Autodesk Fusion 360 part; units mm, degrees
note: some values were not read from the file. Set by a fixed rule: which face or edge a step refers to.
(part 2 of 3)
sketch "Joins" plane through (0, 0, 0) normal (0, 0, 1) x (1, 0, 0)
  line L0 (-32.0183, 52.9002) -> (-40.0183, 52.8995)
  arc A0 (-40.0183, 52.8995) -> (-40.0176, 45.3995) centre (-40.018, 49.1495) ccw
  line L1 (-40.0176, 45.3995) -> (-32.0176, 45.4002)
  arc A1 (-32.0176, 45.4002) -> (-32.0183, 52.9002) centre (-32.018, 49.1502) ccw
  line L2 (-32.018, 49.1502) -> (-40.018, 49.1495) construction
  line L3 (-23.6888, 49.151) -> (-32.018, 49.1502)
  arc A2 (-40.0183, 42.8995) -> (-40.0176, 35.3995) centre (-40.018, 39.1495) ccw
  line L4 (-40.0176, 35.3995) -> (-32.0176, 35.4002)
  arc A3 (-32.0176, 35.4002) -> (-32.0183, 42.9002) centre (-32.018, 39.1502) ccw
  line L5 (-32.0183, 42.9002) -> (-40.0183, 42.8995)
  arc A4 (-32.0176, 25.4002) -> (-32.0183, 32.9002) centre (-32.018, 29.1502) ccw
  line L6 (-32.0183, 32.9002) -> (-40.0183, 32.8995)
  arc A5 (-40.0183, 32.8995) -> (-40.0176, 25.3995) centre (-40.018, 29.1495) ccw
  line L7 (-40.0176, 25.3995) -> (-32.0176, 25.4002)
  arc A6 (-40.0183, 22.8995) -> (-40.0176, 15.3995) centre (-40.018, 19.1495) ccw
  line L8 (-40.0176, 15.3995) -> (-32.0176, 15.4002)
  arc A7 (-32.0176, 15.4002) -> (-32.0183, 22.9002) centre (-32.018, 19.1502) ccw
  line L9 (-32.0183, 22.9002) -> (-40.0183, 22.8995)
  arc A8 (-40.0183, 12.8995) -> (-40.0176, 5.3995) centre (-40.018, 9.1495) ccw
  line L10 (-40.0176, 5.3995) -> (-32.0176, 5.4002)
  arc A9 (-32.0176, 5.4002) -> (-32.0183, 12.9002) centre (-32.018, 9.1502) ccw
  line L11 (-32.0183, 12.9002) -> (-40.0183, 12.8995)
  arc A10 (11.7309, 47.7843) -> (11.9097, 40.2864) centre (11.8203, 44.0353) ccw
  line L12 (11.9097, 40.2864) -> (19.9074, 40.4771)
  arc A11 (19.9074, 40.4771) -> (19.7286, 47.975) centre (19.818, 44.2261) ccw
  line L13 (19.7286, 47.975) -> (11.7309, 47.7843)
  line L14 (11.9129, 30.2801) -> (19.9104, 30.4772)
  arc A12 (19.9104, 30.4772) -> (19.7256, 37.9749) centre (19.818, 34.2261) ccw
  arc A13 (11.7281, 37.7778) -> (11.9129, 30.2801) centre (11.8205, 34.029) ccw
  line L15 (19.7256, 37.9749) -> (11.7281, 37.7778)
  line L16 (11.8351, 20.44) -> (19.835, 20.4761)
  arc A14 (19.835, 20.4761) -> (19.8011, 27.976) centre (19.818, 24.2261) ccw
  arc A15 (11.8012, 27.9399) -> (11.8351, 20.44) centre (11.8181, 24.1899) ccw
  line L17 (19.8011, 27.976) -> (11.8012, 27.9399)
  point P0 (-32.018, 49.1502)
  dimension "d51" = 8
  dimension "d52" = 7.5
  dimension "d53" = 8
  dimension "d54" = 7.5
  dimension "d55" = 8
  dimension "d56" = 7.5
  dimension "d57" = 8
  dimension "d58" = 7.5
  dimension "d59" = 8
  dimension "d60" = 7.5
  dimension "d61" = 8
  dimension "d62" = 7.5
  dimension "d63" = 8
  dimension "d64" = 7.5
  dimension "d65" = 8
  dimension "d66" = 7.5
  constraint tangent L0 A0
  constraint tangent A0 L1
  constraint parallel L0 L1
  constraint tangent L1 A1
  constraint tangent L0 A1
  constraint parallel L2 L3
  constraint coincident P0 A1.centre
  constraint tangent A2 L5
  constraint tangent A2 L4
  constraint parallel L4 L5
  constraint tangent L4 A3
  constraint tangent A3 L5
  constraint tangent L6 A5
  constraint tangent A5 L7
  constraint parallel L6 L7
  constraint tangent A4 L7
  constraint tangent A4 L6
  constraint tangent A6 L9
  constraint tangent A6 L8
  constraint parallel L8 L9
  constraint tangent L8 A7
  constraint tangent A7 L9
  constraint tangent A8 L11
  constraint tangent A8 L10
  constraint parallel L10 L11
  constraint tangent L10 A9
  constraint tangent A9 L11
  constraint tangent A10 L13
  constraint tangent A10 L12
  constraint parallel L12 L13
  constraint tangent L12 A11
  constraint tangent A11 L13
  constraint tangent A13 L15
  constraint tangent L14 A13
  constraint parallel L14 L15
  constraint tangent L14 A12
  constraint tangent A12 L15
  constraint tangent A15 L17
  constraint tangent L16 A15
  constraint parallel L16 L17
  constraint tangent L16 A14
  constraint tangent A14 L17
  measures "d51" distance of P0 A0.centre
  measures "d52" diameter of A0
  measures "d53" distance of A2.centre A3.centre
  measures "d54" diameter of A2
  measures "d55" distance of A5.centre A4.centre
  measures "d56" diameter of A5
  measures "d57" distance of A6.centre A7.centre
  measures "d58" diameter of A6
  measures "d59" distance of A8.centre A9.centre
  measures "d60" diameter of A8
  measures "d61" distance of A10.centre A11.centre
  measures "d62" diameter of A10
  measures "d63" distance of A13.centre A12.centre
  measures "d64" diameter of A13
  measures "d65" distance of A15.centre A14.centre
  measures "d66" diameter of A15
extrude "Extrude8" cut sketch "Joins" against normal blind 2.7 bodies 1
extrude "Extrude9" add sketch "Joins" along normal blind 4 separate body makes body 19 at (-34.6848, 40.4, 0) makes body 20 at (-34.6848, 20.4, 0) makes body 21 at (17.1819, 42.9128, 0) makes body 22 at (-34.6848, 30.4, 0) makes body 23 at (-37.3512, 47.8997, 4) makes body 24 at (-34.6848, 10.4, 0) makes body 25 at (17.1214, 35.41, 0) makes body 26 at (17.1458, 25.464, 0)
move_body "Move4" bodies 22 23 24 21 25 20 26 19 to x (1, 0, 0) y (0, 1, 0) z (0, 0, 1) at (0, 0, -8.7)
combine "Combine5" operation cut target body 1 tool bodies 19 22 25 20 23 24 26 21
sketch "Border" plane through (0, 0, 0) normal (0, 0, 1) x (-1, 0, 0)
  line L0 (101.7185, 44.7509) -> (-98.6412, 44.7509)
  line L1 (-98.6412, 44.7509) -> (-98.6412, -80.6951)
  line L2 (-98.6412, -80.6951) -> (101.7185, -80.6951)
  line L3 (101.7185, -80.6951) -> (101.7185, 44.7509)
  arc A0 (32.0176, -5.4002) -> (28.6259, -7.5514) centre (32.018, -9.1502) ccw
  line L4 (32.0176, -5.4002) -> (40.0176, -5.3995)
  arc A1 (40.0183, -12.8995) -> (40.0176, -5.3995) centre (40.018, -9.1495) ccw
  line L5 (40.0183, -12.8995) -> (32.0183, -12.9002)
  arc A2 (28.6396, -10.7778) -> (32.0183, -12.9002) centre (32.018, -9.1502) ccw
  line L6 (28.6396, -10.7778) -> (26.121, -10.7778)
  line L7 (26.121, -10.7778) -> (26.121, -18.6304)
  arc A3 (24.5959, -20.7696) -> (26.121, -18.6304) centre (24.596, -19.1564) ccw
  line L8 (24.5959, -20.7696) -> (17.0179, -20.7691)
  line L9 (16.4913, -20.6807) -> (2.5732, -20.6743)
  arc A4 (2.5746, -17.6243) -> (2.5732, -20.6743) centre (2.5739, -19.1493) ccw
  line L10 (2.5746, -17.6243) -> (16.4927, -17.6307)
  line L11 (17.0181, -17.5428) -> (23.071, -17.5432)
  line L12 (23.071, -17.5432) -> (23.071, -9.6906)
  arc A5 (24.596, -7.5514) -> (23.071, -9.6906) centre (24.596, -9.1646) ccw
  line L13 (24.596, -7.5514) -> (28.6259, -7.5514)
  circle A6 centre (1.524, -36.656) radius 0.45
  circle A7 centre (17.018, -6.656) radius 0.45
  circle A8 centre (9.271, -0.998) radius 0.45
  circle A9 centre (17.018, -31.656) radius 0.45
  circle A10 centre (17.018, -34.156) radius 0.45
  circle A11 centre (17.018, -9.156) radius 0.45
  circle A12 centre (17.018, -16.656) radius 0.45
  circle A13 centre (1.524, -6.656) radius 0.45
  circle A14 centre (17.018, -26.656) radius 0.45
  circle A15 centre (1.524, -21.656) radius 0.45
  circle A16 centre (1.524, -26.656) radius 0.45
  circle A17 centre (1.524, -9.156) radius 0.45
  circle A18 centre (1.524, -16.656) radius 0.45
  circle A19 centre (9.271, -3) radius 0.45
  circle A20 centre (7.271, -0.9961) radius 0.45
  circle A21 centre (17.018, -4.156) radius 0.45
  circle A22 centre (1.524, -4.156) radius 0.45
  circle A23 centre (11.269, -3) radius 0.45
  circle A24 centre (1.524, -31.656) radius 0.45
  circle A25 centre (1.524, -11.656) radius 0.45
  circle A26 centre (17.018, -21.656) radius 0.45
  circle A27 centre (17.018, -11.656) radius 0.45
  circle A28 centre (17.018, -14.156) radius 0.45
  circle A29 centre (17.018, -36.656) radius 0.45
  circle A30 centre (11.2599, -1.0002) radius 0.45
  circle A31 centre (7.271, -3.0017) radius 0.45
  arc A32 (40.0183, -22.8995) -> (40.0176, -15.3995) centre (40.018, -19.1495) ccw
  line L14 (40.0183, -22.8995) -> (32.0183, -22.9002)
  arc A33 (32.0176, -15.4002) -> (32.0183, -22.9002) centre (32.018, -19.1502) ccw
  line L15 (32.0176, -15.4002) -> (40.0176, -15.3995)
  arc A34 (-11.7309, -47.7843) -> (-11.9097, -40.2864) centre (-11.8203, -44.0353) ccw
  line L16 (-11.7309, -47.7843) -> (-19.7286, -47.975)
  arc A35 (-19.9074, -40.4771) -> (-19.7286, -47.975) centre (-19.818, -44.2261) ccw
  line L17 (-19.9074, -40.4771) -> (-11.9097, -40.2864)
  line L18 (40.0183, -52.8995) -> (32.0183, -52.9002)
  arc A36 (32.0176, -45.4002) -> (32.0183, -52.9002) centre (32.018, -49.1502) ccw
  line L19 (32.0176, -45.4002) -> (40.0176, -45.3995)
  arc A37 (40.0183, -52.8995) -> (40.0176, -45.3995) centre (40.018, -49.1495) ccw
  arc A38 (28.594, -40.6795) -> (32.0183, -42.9002) centre (32.018, -39.1502) ccw
  line L20 (28.594, -40.6795) -> (17.0182, -40.681)
  arc A39 (17.0041, -40.681) -> (17.0182, -40.681) centre (17.018, -39.156) ccw
  line L21 (17.0041, -40.681) -> (1.6701, -40.6778)
  arc A40 (1.6707, -37.6278) -> (1.6701, -40.6778) centre (1.6704, -39.1528) ccw
  line L22 (1.6707, -37.6278) -> (17.0047, -37.631)
  arc A41 (17.0178, -37.6309) -> (17.0047, -37.631) centre (17.018, -39.156) ccw
  line L23 (17.0178, -37.6309) -> (28.5902, -37.6293)
  arc A42 (32.0176, -35.4002) -> (28.5902, -37.6293) centre (32.018, -39.1502) ccw
  line L24 (32.0176, -35.4002) -> (40.0176, -35.3995)
  arc A43 (40.0183, -42.8995) -> (40.0176, -35.3995) centre (40.018, -39.1495) ccw
  line L25 (40.0183, -42.8995) -> (32.0183, -42.9002)
  arc A44 (-8.4113, -22.6228) -> (-11.8351, -20.44) centre (-11.8181, -24.1899) ccw
  line L26 (-8.4113, -22.6228) -> (1.6713, -22.6262)
  line L27 (1.6713, -22.6262) -> (17.0185, -22.631)
  arc A45 (17.0175, -25.681) -> (17.0185, -22.631) centre (17.018, -24.156) ccw
  line L28 (17.0175, -25.681) -> (1.6704, -25.6762)
  line L29 (1.6704, -25.6762) -> (-8.3738, -25.6728)
  line L30 (-11.8012, -27.9399) -> (-19.8011, -27.976)
  arc A46 (-19.835, -20.4761) -> (-19.8011, -27.976) centre (-19.818, -24.2261) ccw
  line L31 (-19.835, -20.4761) -> (-11.8351, -20.44)
  arc A47 (28.596, -30.684) -> (32.0183, -32.9002) centre (32.018, -29.1502) ccw
  line L32 (28.596, -30.684) -> (17.0369, -30.6809)
  arc A48 (17.0176, -30.681) -> (17.0369, -30.6809) centre (17.018, -29.156) ccw
  line L33 (17.0176, -30.681) -> (1.6701, -30.6768)
  arc A49 (1.671, -27.6268) -> (1.6701, -30.6768) centre (1.6705, -29.1518) ccw
  line L34 (1.671, -27.6268) -> (17.0184, -27.631)
  arc A50 (17.0377, -27.6311) -> (17.0184, -27.631) centre (17.018, -29.156) ccw
  line L35 (17.0377, -27.6311) -> (28.5881, -27.6343)
  arc A51 (32.0176, -25.4002) -> (28.5881, -27.6343) centre (32.018, -29.1502) ccw
  line L36 (32.0176, -25.4002) -> (40.0176, -25.3995)
  arc A52 (40.0183, -32.8995) -> (40.0176, -25.3995) centre (40.018, -29.1495) ccw
  line L37 (40.0183, -32.8995) -> (32.0183, -32.9002)
  arc A53 (-8.3422, -32.6274) -> (-11.9129, -30.2801) centre (-11.8205, -34.029) ccw
  line L38 (-8.3422, -32.6274) -> (1.6714, -32.6293)
  line L39 (1.6714, -32.6293) -> (11.7302, -32.631)
  arc A54 (13.1178, -34.7881) -> (11.7302, -32.631) centre (11.73, -34.156) ccw
  arc A55 (10.226, -35.6807) -> (13.1178, -34.7881) centre (11.7277, -35.4153) ccw
  line L40 (10.226, -35.6807) -> (1.6709, -35.6793)
  line L41 (1.6709, -35.6793) -> (-8.4522, -35.6774)
  line L42 (-11.7281, -37.7778) -> (-19.7256, -37.9749)
  arc A56 (-19.9104, -30.4772) -> (-19.7256, -37.9749) centre (-19.818, -34.2261) ccw
  line L43 (-19.9104, -30.4772) -> (-11.9129, -30.2801)
  line L44 (-6.5778, -60.1235) -> (22.1197, -60.1235)
  line L45 (39.1197, -43.1235) -> (39.1197, -2.2457)
  line L46 (26.1197, 10.7543) -> (-6.5778, 10.7543)
  line L47 (-19.5778, -2.2457) -> (-19.5778, -47.1235)
  arc A57 (22.1197, -60.1235) -> (39.1197, -43.1235) centre (22.1197, -43.1235) ccw
  arc A58 (-19.5778, -47.1235) -> (-6.5778, -60.1235) centre (-6.5778, -47.1235) ccw
  arc A59 (39.1197, -2.2457) -> (26.1197, 10.7543) centre (26.1197, -2.2457) ccw
  arc A60 (-6.5778, 10.7543) -> (-19.5778, -2.2457) centre (-6.5778, -2.2457) ccw
  arc A61 (16.4913, -20.6807) -> (17.0179, -20.7691) centre (17.018, -19.156) ccw
  arc A62 (17.0181, -17.5428) -> (16.4927, -17.6307) centre (17.018, -19.156) ccw
  arc A63 (-11.8012, -27.9399) -> (-8.3738, -25.6728) centre (-11.8181, -24.1899) ccw
  arc A64 (-11.7281, -37.7778) -> (-8.4522, -35.6774) centre (-11.8205, -34.029) ccw
  circle A65 centre (1.524, -14.156) radius 0.45
  point P0 (9.271, -24.6846)
  dimension "d76" = 17
  dimension "d77" = 13
  constraint horizontal L44
  constraint perpendicular L44 L45
  constraint parallel L44 L46
  constraint parallel L45 L47
  constraint tangent L45 A57
  constraint tangent L44 A57
  constraint tangent L44 A58
  constraint tangent L47 A58
  constraint tangent L46 A59
  constraint tangent L45 A59
  constraint equal A58 A59
  constraint tangent L46 A60
  constraint tangent L47 A60
  constraint equal A58 A60
  measures "d76" radius of A57
  measures "d77" radius of A58
extrude "Extrude10" cut sketch "Border" against normal blind 8.7 contours A0 L4 L5 A2 L6 L7 A3 L8 L9 A4 L10 L11 L12 A5 L13 L45 A61 A62 | A0 L4 L5 A2 L6 L7 A3 L8 L9 A4 L10 L11 L12 A5 L13 L14 A33 L15 A34 L16 L17 L18 A36 L19 A38 L20 A39 L21 A40 L22 A41 L23 A42 L24 L25 A44 L26 L27 A45 L28 L29 L30 L31 A47 L32 A48 L33 A49 L34 A50 L35 A51 L36 L37 A53 L38 L39 A54 A55 L40 L41 L42 L43 L44 L45 L46 L47 A57 A58 A59 A60 A61 A62 A63 A64 | L4 A1 L5 L45 | L14 A33 L15 L45 | A32 L14 L15 L45 | A47 L32 A48 L33 A49 L34 A50 L35 A51 L36 L37 L45 | L36 A52 L37 L45 | L30 A46 L31 L47 | A44 L26 L27 A45 L28 L29 L30 L31 L47 A63 | A38 L20 A39 L21 A40 L22 A41 L23 A42 L24 L25 L45 | L24 A43 L25 L45 | L42 A56 L43 L47 | A53 L38 L39 A54 A55 L40 L41 L42 L43 L47 A64 | L18 A36 L19 A57 | L18 L19 A37 A57 | L16 A35 L17 L47 A58 | A34 L16 L17 L47 A58 | A6 | A7 | A8 | A9 | A10 | A11 | A12 | A13 | A14 | A15 | A16 | A17 | A18 | A19 | A20 | A21 | A22 | A23 | A24 | A25 | A26 | A27 | A28 | A29 | A30 | A31 | A65 keep common part bodies 1
sketch "ArduinoExtrusion" plane through (0, 0, 0) normal (0, 0, 1) x (1, 0, 0)
  line L0 (-18.542, 0) -> (0, 0)
  line L1 (0, 0) -> (0, 43.18)
  line L2 (0, 43.18) -> (-18.542, 43.18)
  line L3 (-18.542, 43.18) -> (-18.542, 0)
  line L4 (-15.829, 4.2) -> (-2.8014, 4.2)
  line L5 (-2.8014, 4.2) -> (-2.8014, 43.18)
  line L6 (-2.8014, 43.18) -> (-15.829, 43.18)
  line L7 (-15.829, 43.18) -> (-15.829, 4.2)
  line L8 (-15.829, 43.18) -> (-2.8014, 43.18)
  line L9 (-2.8014, 43.18) -> (-2.8014, 65.9759)
  line L10 (-2.8014, 65.9759) -> (-15.829, 65.9759)
  line L11 (-15.829, 65.9759) -> (-15.829, 43.18)
  line L12 (-19.542, -1) -> (1, -1)
  line L13 (1, -1) -> (1, 44.18)
  line L14 (1, 44.18) -> (-19.542, 44.18)
  line L15 (-19.542, 44.18) -> (-19.542, -1)
  point P0 (-18.542, 0)
  point P1 (0, 43.18)
  point P2 (-15.829, 4.2)
  point P3 (-2.8014, 43.18)
  dimension "d92" = 1
  constraint horizontal L0
  constraint vertical L1
  constraint horizontal L2
  constraint vertical L3
  constraint coincident P1 L1.end
  constraint coincident P0 L0.start
  constraint horizontal L4
  constraint vertical L5
  constraint horizontal L6
  constraint vertical L7
  constraint coincident P3 L5.end
  constraint coincident P2 L4.start
  constraint horizontal L8
  constraint vertical L9
  constraint horizontal L10
  constraint vertical L11
extrude "Extrude12" cut sketch "ArduinoExtrusion" against normal blind 0.2 contours L2 L6 L8 L9 L11 L14 | L9 L10 L11 L14 bodies 1
extrude "Extrude13" cut sketch "ArduinoExtrusion" against normal blind 1.2 contours L0 L1 L2 L3 L4 L5 L7 | L0 L1 L2 L3 L9 L11 L12 L13 L14 L15 | L2 L6 L8 L9 L11 L14 | L2 L4 L5 L6 L7 L8 bodies 1
sketch "PaintJointsHole" plane through (0, 0, 0) normal (0, 0, 1) x (1, 0, 0)
  circle A0 centre (-32.018, 49.1502) radius 1.525
  circle A1 centre (-32.018, 39.1502) radius 1.525
  circle A2 centre (-32.018, 29.1502) radius 1.525
  circle A3 centre (-32.018, 19.1502) radius 1.525
  circle A4 centre (-32.018, 9.1502) radius 1.525
  circle A5 centre (11.8181, 24.1899) radius 1.525
  circle A6 centre (11.8205, 34.029) radius 1.525
  circle A7 centre (11.8203, 44.0353) radius 1.525
  point P0 (-32.018, 49.1502)
  point P1 (-32.018, 39.1502)
  point P2 (-32.018, 29.1502)
  point P3 (-32.018, 19.1502)
  point P4 (-32.018, 9.1502)
  point P5 (11.5344, 13.9344)
  point P6 (11.8181, 24.1899)
  point P7 (11.8205, 34.029)
  point P8 (11.8203, 44.0353)
  dimension "d88" = 3.05
  constraint coincident P0 A0.centre
  constraint coincident P1 A1.centre
  constraint coincident P2 A2.centre
  constraint coincident P3 A3.centre
  constraint coincident P4 A4.centre
  constraint coincident P6 A5.centre
  constraint coincident P7 A6.centre
  constraint coincident P8 A7.centre
  constraint equal A0 A1
  constraint equal A0 A2
  constraint equal A0 A7
  constraint equal A0 A6
  constraint equal A0 A5
  constraint equal A0 A3
  constraint equal A0 A4
  measures "d88" diameter of A0
extrude "Extrude15" cut sketch "PaintJointsHole" against normal blind 8.7 bodies 1
sketch "CutBetweenLeg" plane through (0, 0, 0) normal (0, 0, 1) x (1, 0, 0)
  line L0 (-39.1197, 35.6745) -> (-53.3111, 35.6745)
  arc A0 (-53.3111, 35.6745) -> (-53.3111, 32.6245) centre (-53.3111, 34.1495) ccw
  line L1 (-53.3111, 32.6245) -> (-39.1197, 32.6245)
  arc A1 (-39.1197, 32.6245) -> (-39.1197, 35.6745) centre (-39.1197, 34.1495) ccw
  line L2 (-39.1197, 34.1495) -> (-53.3111, 34.1495) construction
  line L3 (-39.1197, 32.8995) -> (-39.1197, 35.3995)
  line L4 (-39.0814, 45.7891) -> (-53.3111, 45.7891)
  arc A2 (-53.3111, 45.7891) -> (-53.3111, 42.7391) centre (-53.3111, 44.2641) ccw
  line L5 (-53.3111, 42.7391) -> (-39.0814, 42.7391)
  arc A3 (-39.0814, 42.7391) -> (-39.0814, 45.7891) centre (-39.0814, 44.2641) ccw
  line L6 (-39.0814, 44.2641) -> (-53.3111, 44.2641) construction
  arc A4 (-38.9667, 45.3996) -> (-39.1197, 43.1235) centre (-22.1197, 43.1235) ccw
  line L7 (-39.1197, 25.6745) -> (-53.3111, 25.6745)
  arc A5 (-53.3111, 25.6745) -> (-53.3111, 22.6245) centre (-53.3111, 24.1495) ccw
  line L8 (-53.3111, 22.6245) -> (-39.1197, 22.6245)
  arc A6 (-39.1197, 22.6245) -> (-39.1197, 25.6745) centre (-39.1197, 24.1495) ccw
  line L9 (-39.1197, 24.1495) -> (-53.3111, 24.1495) construction
  line L10 (-39.1197, 22.8995) -> (-39.1197, 25.3995)
  line L11 (-39.1197, 15.6745) -> (-53.3111, 15.6745)
  arc A7 (-53.3111, 15.6745) -> (-53.3111, 12.6245) centre (-53.3111, 14.1495) ccw
  line L12 (-53.3111, 12.6245) -> (-39.1197, 12.6245)
  arc A8 (-39.1197, 12.6245) -> (-39.1197, 15.6745) centre (-39.1197, 14.1495) ccw
  line L13 (-39.1197, 14.1495) -> (-53.3111, 14.1495) construction
  line L14 (-39.1197, 12.8995) -> (-39.1197, 15.3995)
  line L15 (19.5778, 20.4749) -> (19.5778, 2.2457)
  line L16 (19.5778, 27.697) -> (37.3869, 27.697)
  arc A9 (37.3869, 27.697) -> (37.3869, 30.747) centre (37.3869, 29.222) ccw
  line L17 (37.3869, 30.747) -> (19.5778, 30.747)
  arc A10 (19.5778, 30.747) -> (19.5778, 27.697) centre (19.5778, 29.222) ccw
  line L18 (19.5778, 29.222) -> (37.3869, 29.222) construction
  line L19 (19.5778, 30.469) -> (19.5778, 27.975)
  line L20 (19.5778, 37.6953) -> (37.3869, 37.6953)
  arc A11 (37.3869, 37.6953) -> (37.3869, 40.7453) centre (37.3869, 39.2203) ccw
  line L21 (37.3869, 40.7453) -> (19.5778, 40.7453)
  arc A12 (19.5778, 40.7453) -> (19.5778, 37.6953) centre (19.5778, 39.2203) ccw
  line L22 (19.5778, 39.2203) -> (37.3869, 39.2203) construction
  line L23 (19.5778, 40.4693) -> (19.5778, 37.9713)
  dimension "d108" = 3.05
  dimension "d109" = 3.05
  dimension "d110" = 3.05
  dimension "d111" = 3.05
  dimension "d113" = 3.05
  dimension "d114" = 3.05
  constraint tangent L0 A0
  constraint tangent A0 L1
  constraint parallel L0 L1
  constraint tangent L1 A1
  constraint tangent L0 A1
  constraint perpendicular L2 L3
  constraint midpoint A1.centre L3
  constraint tangent L4 A2
  constraint tangent A2 L5
  constraint parallel L4 L5
  constraint tangent L5 A3
  constraint tangent L4 A3
  constraint parallel L0 L6
  constraint midpoint A3.centre A4
  constraint tangent L7 A5
  constraint tangent A5 L8
  constraint parallel L7 L8
  constraint tangent L8 A6
  constraint tangent L7 A6
  constraint perpendicular L3 L9
  constraint midpoint A6.centre L10
  constraint tangent L11 A7
  constraint tangent A7 L12
  constraint parallel L11 L12
  constraint tangent L12 A8
  constraint tangent L11 A8
  constraint perpendicular L13 L14
  constraint midpoint A8.centre L14
  constraint tangent L16 A9
  constraint tangent A9 L17
  constraint parallel L16 L17
  constraint tangent L17 A10
  constraint tangent L16 A10
  constraint perpendicular L18 L19
  constraint midpoint A10.centre L19
  constraint tangent L20 A11
  constraint tangent A11 L21
  constraint parallel L20 L21
  constraint tangent L21 A12
  constraint tangent L20 A12
  constraint perpendicular L22 L23
  constraint midpoint A12.centre L23
  measures "d108" diameter of A0
  measures "d109" diameter of A2
  measures "d110" diameter of A5
  measures "d111" diameter of A7
  measures "d113" diameter of A9
  measures "d114" diameter of A11
extrude "Extrude17" cut sketch "CutBetweenLeg" against normal blind 8.7 bodies 1
sketch "Sketch20" plane through (0, 0, 0) normal (0, 0, 1) x (1, 0, 0)
  line L0 (21.2354, 40.7542) -> (19.5778, 40.7508)
  line L1 (19.5778, 37.7008) -> (21.2402, 37.6959)
  arc A0 (18.7043, 37.9757) -> (19.5778, 37.7008) centre (19.5778, 39.2258) ccw
  arc A1 (18.7041, 40.4757) -> (18.7043, 37.9757) centre (19.5778, 39.2258) ccw
  arc A2 (19.5778, 40.7508) -> (18.7041, 40.4757) centre (19.5778, 39.2258) ccw
  line L2 (21.2434, 20.7575) -> (19.5778, 20.7508)
  line L3 (19.5778, 17.7008) -> (21.251, 17.6915)
  arc A3 (18.7043, 17.9757) -> (19.5778, 17.7008) centre (19.5778, 19.2258) ccw
  arc A4 (18.7041, 20.4757) -> (18.7043, 17.9757) centre (19.5778, 19.2258) ccw
  arc A5 (19.5778, 20.7508) -> (18.7041, 20.4757) centre (19.5778, 19.2258) ccw
  line L4 (-41.123, 42.732) -> (-39.0815, 42.7388)
  arc A6 (-38.0632, 45.3991) -> (-39.0815, 45.7888) centre (-39.0815, 44.2638) ccw
  arc A7 (-38.401, 42.899) -> (-38.0632, 45.3991) centre (-39.0815, 44.2638) ccw
  arc A8 (-39.0815, 42.7388) -> (-38.401, 42.899) centre (-39.0815, 44.2638) ccw
  line L5 (-39.0815, 45.7888) -> (-41.6972, 45.7955)
  line L6 (-41.4536, 12.6128) -> (-39.1197, 12.624)
  line L7 (-39.1197, 15.674) -> (-41.4536, 15.6842)
  arc A9 (-38.2463, 15.3991) -> (-39.1197, 15.674) centre (-39.1197, 14.149) ccw
  arc A10 (-38.2461, 12.8991) -> (-38.2463, 15.3991) centre (-39.1197, 14.149) ccw
  arc A11 (-39.1197, 12.624) -> (-38.2461, 12.8991) centre (-39.1197, 14.149) ccw
  line L8 (-41.4513, 22.6138) -> (-39.1197, 22.624)
  line L9 (-39.1197, 25.674) -> (-41.4504, 25.6829)
  arc A12 (-38.2463, 25.3991) -> (-39.1197, 25.674) centre (-39.1197, 24.149) ccw
  arc A13 (-38.2461, 22.8991) -> (-38.2463, 25.3991) centre (-39.1197, 24.149) ccw
  arc A14 (-39.1197, 22.624) -> (-38.2461, 22.8991) centre (-39.1197, 24.149) ccw
  line L10 (21.2387, 30.7556) -> (19.5778, 30.7508)
  line L11 (19.5778, 27.7008) -> (21.245, 27.694)
  arc A15 (18.7043, 27.9757) -> (19.5778, 27.7008) centre (19.5778, 29.2258) ccw
  arc A16 (18.7041, 30.4757) -> (18.7043, 27.9757) centre (19.5778, 29.2258) ccw
  arc A17 (19.5778, 30.7508) -> (18.7041, 30.4757) centre (19.5778, 29.2258) ccw
  line L12 (-41.4481, 32.6151) -> (-39.1197, 32.624)
  line L13 (-39.1197, 35.674) -> (-41.4471, 35.6815)
  arc A18 (-38.2463, 35.3991) -> (-39.1197, 35.674) centre (-39.1197, 34.149) ccw
  arc A19 (-38.2461, 32.8991) -> (-38.2463, 35.3991) centre (-39.1197, 34.149) ccw
  arc A20 (-39.1197, 32.624) -> (-38.2461, 32.8991) centre (-39.1197, 34.149) ccw
  arc A21 (21.2354, 40.7542) -> (19.8553, 47.9759) centre (19.818, 44.2261) ccw
  line L14 (19.8553, 47.9759) -> (19.5498, 47.9758)
  arc A22 (-41.4536, 12.6128) -> (-40.1195, 5.3999) centre (-40.018, 9.1485) ccw
  line L15 (-40.1195, 5.3999) -> (-39.1197, 5.399)
  arc A23 (21.2434, 20.7575) -> (21.245, 27.694) centre (19.818, 24.2261) ccw
  arc A24 (-41.123, 42.732) -> (-41.4471, 35.6815) centre (-40.018, 39.1485) ccw
  arc A25 (21.2387, 30.7556) -> (21.2402, 37.6959) centre (19.818, 34.2261) ccw
  arc A26 (-40.0187, 52.8985) -> (-41.6972, 45.7955) centre (-40.018, 49.1485) ccw
  line L16 (19.5778, 10.4758) -> (19.6718, 10.4789)
  arc A27 (19.5498, 47.9758) -> (6.5778, 60.1235) centre (6.5778, 47.1235) ccw
  line L17 (6.5778, 60.1235) -> (-21.2217, 60.1235)
  arc A28 (-21.2217, 60.1235) -> (-36.0278, 52.8993) centre (-22.1037, 43.1464) ccw
  arc A29 (-41.4481, 32.6151) -> (-41.4504, 25.6829) centre (-40.018, 29.1485) ccw
  arc A30 (-41.4513, 22.6138) -> (-41.4536, 15.6842) centre (-40.018, 19.1485) ccw
  line L18 (-39.1197, 5.399) -> (-39.1197, 2.2457)
  arc A31 (-39.1197, 2.2457) -> (-27.0619, -10.7543) centre (-26.1198, 2.2115) ccw
  line L19 (-27.0619, -10.7543) -> (6.5778, -10.7543)
  arc A32 (6.5778, -10.7543) -> (19.5778, 2.2457) centre (6.5778, 2.2457) ccw
  line L20 (19.5778, 2.2457) -> (19.5778, 10.4758)
  arc A33 (19.6718, 10.4789) -> (21.251, 17.6915) centre (19.818, 14.2261) ccw
  line L21 (-36.0278, 52.8993) -> (-40.0187, 52.8985)
  constraint tangent A26 L21
sketch "Sketch21" plane through (0, 0, 0) normal (0, 0, 1) x (1, 0, 0)
sketch "Sketch22" plane through (0, 0, 0) normal (0, 0, 1) x (1, 0, 0)
sketch "BluetoothJointsPath" plane through (0, 0, 0) normal (0, 0, 1) x (1, 0, 0)
  circle A0 centre (-1.524, 16.656) radius 0.45
  line L0 (-1.524, 16.656) -> (13.563, 16.656) construction
  line L1 (13.563, 16.656) -> (13.563, -3.0633) construction
  circle A1 centre (-1.524, 14.156) radius 0.45
  line L2 (-1.524, 14.156) -> (5.5131, 14.156) construction
  line L3 (5.5131, 14.156) -> (5.5131, -3.0633) construction
  circle A2 centre (-1.524, 11.656) radius 0.45
  line L4 (1, 22.6253) -> (1, -1)
  line L5 (-1.524, 11.656) -> (-4.4669, 11.656) construction
  line L6 (-4.4669, 11.656) -> (-4.4669, -3.5542) construction
  circle A3 centre (-17.018, 11.656) radius 0.45
  line L7 (-17.018, 11.656) -> (-13.9546, 11.656) construction
  line L8 (-13.9546, 11.656) -> (-13.9546, -3.7538) construction
  circle A4 centre (-17.018, 4.156) radius 0.45
  line L9 (-19.542, -1) -> (-19.542, 17.543)
  line L10 (-17.018, 4.156) -> (-26.4105, 4.156) construction
  line L11 (1, -1) -> (-19.542, -1)
  line L12 (-26.4105, 4.156) -> (-26.4105, -13.232) construction
  circle A5 centre (-17.018, 6.656) radius 0.45
  line L13 (-17.018, 6.656) -> (-26.4228, 6.656) construction
  line L14 (-26.4228, 6.656) -> (-26.4228, -13.2059) construction
  arc A6 (-39.1197, 2.2457) -> (-26.1197, -10.7543) centre (-26.1197, 2.2457) ccw
  arc A7 (6.5778, -10.7543) -> (19.5778, 2.2457) centre (6.5778, 2.2457) ccw
  line L15 (-35.3121, -6.9467) -> (15.7701, -6.9467) construction
  circle A8 centre (-7.271, 3.0017) radius 0.45
  line L16 (-6.821, 3.0017) -> (-1.974, 3.0017) construction
  circle A9 centre (-1.524, 4.156) radius 0.45
  line L17 (-1.974, 3.0017) -> (-1.974, 4.156) construction
  line L18 (-11.719, 3) -> (-16.568, 3) construction
  line L19 (-16.568, 3) -> (-16.568, 4.156) construction
  line L20 (-35.3121, -6.9467) -> (-29.6553, -1.2899)
  line L21 (-35.3121, -6.9467) -> (-27.3121, -6.9467) construction
  point P0 (-1.974, 4.156)
  point P1 (-11.719, 3)
  point P2 (-14.1435, 3)
  point P3 (-4.3975, 3.0017)
  dimension "d147" = 45
  dimension "d148" = 8
  constraint coincident A0.centre L0.start
  constraint horizontal L0
  constraint perpendicular L0 L1
  constraint coincident A1.centre L2.start
  constraint parallel L1 L3
  constraint coincident A2.centre L5.start
  constraint perpendicular L4 L5
  constraint perpendicular L5 L6
  constraint coincident A3.centre L7.start
  constraint horizontal L7
  constraint perpendicular L7 L8
  constraint coincident A4.centre L10.start
  constraint perpendicular L9 L10
  constraint perpendicular L11 L12
  constraint coincident A5.centre L13.start
  constraint horizontal L13
  constraint perpendicular L13 L14
  constraint midpoint A6 L15.start
  constraint midpoint A7 L15.end
  constraint coincident A8 L16.start
  constraint perpendicular L6 L16
  constraint coincident P0 L17.end
  constraint tangent A9 L17
  constraint coincident P1 L18.start
  constraint perpendicular L8 L18
  constraint coincident A4 L19.end
  constraint tangent A4 L19
  constraint perpendicular L18 L19
  constraint perpendicular L16 L17
  constraint midpoint L18 P2
  constraint midpoint L16 P3
  constraint perpendicular L2 L3
  constraint horizontal L21
  measures "d147" angle of L20 L21
  measures "d148" distance of L15.start L20.end
sketch "BluetoothDOwn" plane through (0, 0, 0) normal (0, 0, 1) x (1, 0, 0)
  line L0 (-12.4994, -5.6447) -> (-12.6185, 11.6665)
  arc A0 (-12.6185, 11.6665) -> (-15.6685, 11.656) centre (-14.1435, 11.656) ccw
  line L1 (-15.9066, 11.6439) -> (-15.7875, -5.6673)
  arc A1 (-15.7875, -5.6673) -> (-12.4994, -5.6447) centre (-14.1435, -5.656) ccw
  line L2 (-14.1435, -5.656) -> (-14.1435, 11.656) construction
  line L3 (-17.018, 11.656) -> (-13.9546, 11.656)
  line L4 (-2.8031, -5.6404) -> (-2.942, 11.6682)
  arc A2 (-2.942, 11.6682) -> (-5.9919, 11.6437) centre (-4.4669, 11.656) ccw
  line L5 (-5.9919, 11.6437) -> (-5.853, -5.6649)
  arc A3 (-5.853, -5.6649) -> (-2.8031, -5.6404) centre (-4.328, -5.6526) ccw
  line L6 (-4.328, -5.6526) -> (-4.4669, 11.656) construction
  line L7 (-1.524, 15.131) -> (13.563, 15.131)
  arc A4 (13.563, 15.131) -> (13.563, 18.181) centre (13.563, 16.656) ccw
  line L8 (13.563, 18.181) -> (-1.524, 18.181)
  arc A5 (-1.524, 18.181) -> (-1.524, 15.131) centre (-1.524, 16.656) ccw
  line L9 (-1.524, 16.656) -> (13.563, 16.656) construction
  line L10 (13.563, 16.656) -> (13.563, -3.0633)
  line L11 (-17.018, 6.656) -> (-26.4228, 6.656) construction
  line L12 (-26.4228, 6.656) -> (-26.4228, -13.2059)
  line L13 (-24.0873, 5.131) -> (-18.0017, 5.131)
  arc A6 (-18.0017, 5.131) -> (-18.0017, 8.181) centre (-18.0017, 6.656) ccw
  line L14 (-18.0017, 8.181) -> (-24.0873, 8.181)
  arc A7 (-24.0873, 8.181) -> (-24.0873, 5.131) centre (-24.0873, 6.656) ccw
  line L15 (-24.0873, 6.656) -> (-18.0017, 6.656) construction
  line L16 (-25.6123, 6.656) -> (-25.6123, -6.9467)
  arc A8 (-25.6123, -6.9467) -> (-22.5623, -6.9467) centre (-24.0873, -6.9467) ccw
  line L17 (-22.5623, -6.9467) -> (-22.5623, 6.656)
  arc A9 (-22.5623, 6.656) -> (-25.6123, 6.656) centre (-24.0873, 6.656) ccw
  line L18 (-24.0873, 6.656) -> (-24.0873, -6.9467) construction
  line L19 (-35.3121, -6.9467) -> (15.7701, -6.9467)
  line L20 (12.038, 16.656) -> (12.038, -6.9467)
  arc A10 (12.038, -6.9467) -> (15.088, -6.9467) centre (13.563, -6.9467) ccw
  line L21 (15.088, -6.9467) -> (15.088, 16.656)
  arc A11 (15.088, 16.656) -> (12.038, 16.656) centre (13.563, 16.656) ccw
  line L22 (13.563, 16.656) -> (13.563, -6.9467) construction
  line L23 (-14.154, 13.1809) -> (-15.9171, 13.1688)
  arc A12 (-15.9171, 13.1688) -> (-15.8961, 10.1189) centre (-15.9066, 11.6439) ccw
  line L24 (-15.8961, 10.1189) -> (-14.133, 10.131)
  arc A13 (-14.133, 10.131) -> (-14.154, 13.1809) centre (-14.1435, 11.656) ccw
  line L25 (-14.1435, 11.656) -> (-15.9066, 11.6439) construction
  line L26 (-4.4547, 10.131) -> (-2.6131, 10.1458)
  arc A14 (-2.6131, 10.1458) -> (-2.6376, 13.1957) centre (-2.6254, 11.6708) ccw
  line L27 (-2.6376, 13.1957) -> (-4.4792, 13.1809)
  arc A15 (-4.4792, 13.1809) -> (-4.4547, 10.131) centre (-4.4669, 11.656) ccw
  line L28 (-4.4669, 11.656) -> (-2.6254, 11.6708) construction
  point P0 (-14.1435, 3)
  point P1 (-14.1435, 3)
  point P2 (-4.3975, 3.0017)
  point P3 (-4.3975, 3.0017)
  point P4 (-4.4669, 11.656)
  point P5 (-1.524, 16.656)
  point P6 (13.563, 16.656)
  point P7 (-17.018, 6.656)
  point P8 (-26.4228, 6.656)
  dimension "d127" = 3.05
  dimension "d128" = 3.05
  dimension "d129" = 3.05
  dimension "d131" = 3.05
  dimension "d132" = 3.05
  dimension "d133" = 3.05
  dimension "d134" = 3.05
  dimension "d135" = 3.05
  constraint tangent L0 A0
  constraint parallel L0 L1
  constraint tangent L1 A1
  constraint tangent L0 A1
  constraint coincident A0.centre L3
  constraint perpendicular L2 L3
  constraint coincident P1 P0
  constraint midpoint L2 P1
  constraint tangent L4 A2
  constraint tangent A2 L5
  constraint parallel L4 L5
  constraint tangent L5 A3
  constraint tangent L4 A3
  constraint coincident P4 A2.centre
  constraint coincident P3 P2
  constraint midpoint L6 P3
  constraint tangent A4 L8
  constraint parallel L7 L8
  constraint tangent L8 A5
  constraint tangent L7 A5
  constraint coincident P6 A4.centre
  constraint perpendicular L9 L10
  constraint coincident P5 A5.centre
  constraint coincident P8 L11.end
  constraint perpendicular L11 L12
  constraint coincident P7 L11.start
  constraint tangent L13 A6
  constraint tangent A6 L14
  constraint parallel L13 L14
  constraint tangent L14 A7
  constraint tangent L13 A7
  constraint coincident L11 A6.centre
  constraint coincident L11 A7.centre
  constraint tangent L16 A8
  constraint tangent A8 L17
  constraint parallel L16 L17
  constraint tangent L17 A9
  constraint tangent L16 A9
  constraint coincident A8.centre L19
  constraint perpendicular L11 L18
  constraint coincident A7.centre L15.start
  constraint tangent L20 A10
  constraint tangent A10 L21
  constraint parallel L20 L21
  constraint tangent L21 A11
  constraint tangent L20 A11
  constraint coincident L19 A10.centre
  constraint perpendicular L19 L22
  constraint tangent L23 A12
  constraint tangent A12 L24
  constraint parallel L23 L24
  constraint tangent L24 A13
  constraint tangent L23 A13
  constraint coincident L1.start A12.centre
  constraint perpendicular L1 L25
  constraint coincident A0.centre L2.end
  constraint tangent L26 A14
  constraint tangent A14 L27
  constraint parallel L26 L27
  constraint tangent L27 A15
  constraint tangent L26 A15
  constraint perpendicular L4 L28
  measures "d127" diameter of A0
  measures "d128" diameter of A2
  measures "d129" diameter of A4
  measures "d131" diameter of A6
  measures "d132" diameter of A8
  measures "d133" diameter of A10
  measures "d134" diameter of A12
  measures "d135" diameter of A14
sketch "BluetoothTop" plane through (0, 0, 0) normal (0, 0, 1) x (1, 0, 0)
  line L0 (-17.018, 5.681) -> (-26.4105, 5.681)
  arc A0 (-26.4105, 5.681) -> (-26.4105, 2.631) centre (-26.4105, 4.156) ccw
  line L1 (-26.4105, 2.631) -> (-17.018, 2.631)
  arc A1 (-17.018, 2.631) -> (-17.018, 5.681) centre (-17.018, 4.156) ccw
  line L2 (-17.018, 4.156) -> (-26.4105, 4.156) construction
  line L3 (-26.4105, 4.156) -> (-26.4105, -13.232)
  line L4 (-27.9351, 4.156) -> (-27.9351, -6.9467)
  arc A2 (-27.9351, -6.9467) -> (-24.8858, -6.9467) centre (-26.4105, -6.9467) ccw
  line L5 (-24.8858, -6.9467) -> (-24.8858, 4.156)
  arc A3 (-24.8858, 4.156) -> (-27.9351, 4.156) centre (-26.4105, 4.156) ccw
  line L6 (-26.4105, 4.156) -> (-26.4105, -6.9467) construction
  line L7 (-35.3121, -6.9467) -> (15.7701, -6.9467)
  line L8 (1, 22.6253) -> (1, -1)
  line L9 (-1.524, 12.631) -> (5.5131, 12.631)
  arc A4 (5.5131, 12.631) -> (5.5131, 15.681) centre (5.5131, 14.156) ccw
  line L10 (5.5131, 15.681) -> (-1.524, 15.681)
  arc A5 (-1.524, 15.681) -> (-1.524, 12.631) centre (-1.524, 14.156) ccw
  line L11 (-1.524, 14.156) -> (5.5131, 14.156) construction
  line L12 (3.9881, 14.156) -> (3.9881, -6.9467)
  arc A6 (3.9881, -6.9467) -> (7.0381, -6.9467) centre (5.5131, -6.9467) ccw
  line L13 (7.0381, -6.9467) -> (7.0381, 14.156)
  arc A7 (7.0381, 14.156) -> (3.9881, 14.156) centre (5.5131, 14.156) ccw
  line L14 (5.5131, 14.156) -> (5.5131, -6.9467) construction
  line L15 (5.5131, 12.631) -> (13.563, 12.631)
  arc A8 (13.563, 12.631) -> (13.563, 15.681) centre (13.563, 14.156) ccw
  line L16 (13.563, 15.681) -> (5.5131, 15.681)
  arc A9 (5.5131, 15.681) -> (5.5131, 12.631) centre (5.5131, 14.156) ccw
  line L17 (5.5131, 14.156) -> (13.563, 14.156) construction
  line L18 (13.563, 16.656) -> (13.563, -6.9467)
  circle A10 centre (13.563, 14.156) radius 1.525
  point P0 (-17.018, 4.156)
  point P1 (-26.4105, 4.156)
  point P2 (-1.524, 14.156)
  point P3 (5.5131, 14.156)
  dimension "d136" = 3.05
  dimension "d137" = 3.05
  dimension "d138" = 3.05
  constraint tangent L0 A0
  constraint tangent A0 L1
  constraint parallel L0 L1
  constraint tangent L1 A1
  constraint tangent L0 A1
  constraint coincident P1 A0.centre
  constraint perpendicular L2 L3
  constraint coincident P0 A1.centre
  constraint tangent L4 A2
  constraint tangent A2 L5
  constraint parallel L4 L5
  constraint tangent L5 A3
  constraint tangent L4 A3
  constraint coincident A2.centre L7
  constraint perpendicular L6 L7
  constraint tangent L9 A4
  constraint tangent A4 L10
  constraint parallel L9 L10
  constraint tangent L10 A5
  constraint tangent L9 A5
  constraint coincident P3 A4.centre
  constraint perpendicular L8 L11
  constraint coincident P2 A5.centre
  constraint tangent L12 A6
  constraint tangent A6 L13
  constraint parallel L12 L13
  constraint tangent L13 A7
  constraint tangent L12 A7
  constraint coincident L7 A6.centre
  constraint perpendicular L7 L14
  constraint tangent L15 A8
  constraint tangent A8 L16
  constraint parallel L15 L16
  constraint tangent L16 A9
  constraint tangent L15 A9
  constraint coincident A8.centre L18
  constraint perpendicular L17 L18
  constraint concentric A8 A10
  measures "d136" diameter of A0
  measures "d137" diameter of A4
  measures "d138" diameter of A6
extrude "Extrude20" add sketch "BluetoothDOwn" along normal blind 4 separate body contours L0 L1 A1 L19 L24 A13 | A0 L23 A12 L24 A13 | L4 L5 A3 L19 L26 A15 | L4 A2 L26 A15 | L4 A2 L26 A14 L27 | L7 L8 A5 L20 A11 | L7 A4 L20 A11 | L7 A4 L19 L20 L21 | L19 A10 | L13 A7 L17 A9 | L13 A7 L16 L17 L19 | L13 A6 L14 L17 A9 | A8 L19 makes body 27 at (-5.9456, 5.8742, 1.3333) makes body 28 at (-12.5391, 0.1257, 2.6667) makes body 29 at (14.0714, 8.2801, 0) makes body 30 at (-24.5957, 1.6134, 0)
move_body "Move18" bodies 30 28 27 29 to x (1, 0, 0) y (0, 1, 0) z (0, 0, 1) at (0, 0, -8.7)
combine "Combine6" operation cut target body 1 tool bodies 27 30 28 29
extrude "Extrude21" cut sketch "BluetoothTop" against normal blind 2.7 contours L0 L1 A1 L5 A3 | A0 L1 L5 A3 | A0 L3 L4 L7 | L1 L3 L5 L7 | L3 A2 L7 | L3 A2 L7 | L7 L9 L12 L13 L15 | L7 A6 | L9 L12 A9 | L8 L9 L10 L12 A7 A9 | A4 L13 L15 | A4 L13 A7 L15 L16 A10 | L8 L9 L10 A5 | A4 A7 A9 | A8 L18 A10 | L18 A10 bodies 1
sketch "BluetoothJoints" plane through (0, 0, 0) normal (0, 0, 1) x (1, 0, 0)
  line L0 (-21.3982, -10.9313) -> (-21.4228, -2.9314)
  arc A0 (-21.4228, -2.9314) -> (-31.4228, -2.9621) centre (-26.4228, -2.9467) ccw
  line L1 (-31.4228, -2.9621) -> (-31.3981, -10.9621)
  arc A1 (-31.3981, -10.9621) -> (-21.3982, -10.9313) centre (-26.3982, -10.9467) ccw
  line L2 (-26.3982, -10.9467) -> (-26.4228, -2.9467) construction
  arc A2 (-27.9351, -6.9467) -> (-24.8858, -6.9467) centre (-26.4105, -6.9467) ccw
  line L3 (-26.4228, 6.656) -> (-26.4228, -13.2059)
  line L4 (-17.9647, -6.9763) -> (-17.9401, -10.9763)
  arc A3 (-17.9401, -10.9763) -> (-11.9402, -10.9393) centre (-14.9402, -10.9578) ccw
  line L5 (-11.9402, -10.9393) -> (-11.9649, -6.9394)
  arc A4 (-11.9649, -6.9394) -> (-17.9647, -6.9763) centre (-14.9648, -6.9578) ccw
  line L6 (-8.4647, -6.9763) -> (-8.4401, -10.9763)
  arc A5 (-8.4401, -10.9763) -> (-2.4402, -10.9393) centre (-5.4402, -10.9578) ccw
  line L7 (-2.4402, -10.9393) -> (-2.4649, -6.9394)
  arc A6 (-2.4649, -6.9394) -> (-8.4647, -6.9763) centre (-5.4648, -6.9578) ccw
  arc A7 (1.5599, -10.9763) -> (7.5598, -10.9393) centre (4.5598, -10.9578) ccw
  line L8 (7.5598, -10.9393) -> (7.5351, -6.9394)
  arc A8 (7.5351, -6.9394) -> (1.5353, -6.9763) centre (4.5352, -6.9578) ccw
  line L9 (1.5353, -6.9763) -> (1.5599, -10.9763)
  line L10 (10.5553, -3.9763) -> (10.5799, -7.9763)
  arc A9 (10.5799, -7.9763) -> (16.5798, -7.9393) centre (13.5798, -7.9578) ccw
  line L11 (16.5798, -7.9393) -> (16.5551, -3.9394)
  arc A10 (16.5551, -3.9394) -> (10.5553, -3.9763) centre (13.5552, -3.9578) ccw
  circle A11 centre (-26.4228, -2.9467) radius 5
  line L12 (-31.4104, -8.4714) -> (-21.4058, -8.4406)
  point P0 (-26.4105, -6.9467)
  dimension "d149" = 4
  dimension "d150" = 10
  dimension "d151" = 6
  dimension "d152" = 6
  dimension "d153" = 6
  dimension "d154" = 6
  constraint tangent L0 A0
  constraint tangent A0 L1
  constraint parallel L0 L1
  constraint tangent L1 A1
  constraint tangent L0 A1
  constraint coincident A0.centre L3
  constraint coincident P0 A2.centre
  constraint midpoint L2 P0
  constraint tangent L5 A4
  constraint tangent L4 A4
  constraint parallel L4 L5
  constraint tangent L4 A3
  constraint tangent A3 L5
  constraint tangent L7 A6
  constraint tangent L6 A6
  constraint parallel L6 L7
  constraint tangent L6 A5
  constraint tangent A5 L7
  constraint tangent L8 A8
  constraint tangent A8 L9
  constraint parallel L8 L9
  constraint tangent A7 L9
  constraint tangent A7 L8
  constraint tangent L11 A10
  constraint tangent L10 A10
  constraint parallel L10 L11
  constraint tangent L10 A9
  constraint tangent A9 L11
  constraint concentric A0 A11
  constraint coincident L0 L12.end
  constraint perpendicular L0 L12
  measures "d149" distance of A0.centre P0
  measures "d150" diameter of A0
  measures "d151" diameter of A4
  measures "d152" diameter of A6
  measures "d153" diameter of A8
  measures "d154" diameter of A10
extrude "Extrude22" cut sketch "BluetoothJoints" against normal blind 2.7 bodies 1
extrude "Extrude23" add sketch "BluetoothJoints" along normal blind 4 separate body makes body 31 at (-4.4484, -9.6183, 0) makes body 32 at (-13.9484, -9.6183, 0) makes body 33 at (3.5434, -8.2973, 0) makes body 34 at (-24.7397, -8.2749, 4) makes body 35 at (14.5716, -6.6183, 0)
move_body "Move19" bodies 34 32 31 33 35 to x (1, 0, 0) y (0, 1, 0) z (0, 0, 1) at (0, 0, -8.7)
combine "Combine7" operation cut target body 1 tool bodies 35 33 31 32 34
sketch "Sketch27" plane through (0, 0, 0) normal (0, 0, 1) x (1, 0, 0)
  circle A0 centre (-15.5964, 53.5303) radius 5
  circle A1 centre (-3.9123, 52.1806) radius 4
  dimension "d169" = 10
  dimension "d170" = 8
  measures "d169" diameter of A0
  measures "d170" diameter of A1
extrude "Extrude26" cut sketch "Sketch27" against normal blind 8.7 bodies 1
sketch "Sketch29" plane through (0, 0, 0) normal (0, 0, 1) x (1, 0, 0)
  circle A0 centre (-19.6701, -10.7543) radius 1.7286
  line L0 (-21.3987, -10.7543) -> (-17.9415, -10.7543)
  circle A1 centre (-10.1914, -10.7543) radius 1.7499
  line L1 (-8.4415, -10.7543) -> (-11.9414, -10.7543)
  circle A2 centre (-0.4414, -10.7543) radius 1.9999
  line L2 (-2.4414, -10.7543) -> (1.5585, -10.7543)
  circle A3 centre (9.447, -10.4338) radius 1.9552
  arc A4 (7.5584, -10.7173) -> (11.2737, -9.8766) centre (6.5778, 2.2457) ccw
  circle A5 centre (-14.9648, -6.9578) radius 1.525
  arc A6 (-11.9649, -6.9394) -> (-17.9647, -6.9763) centre (-14.9648, -6.9578) ccw
  circle A7 centre (-5.4648, -6.9578) radius 1.525
  arc A8 (-2.4649, -6.9394) -> (-8.4647, -6.9763) centre (-5.4648, -6.9578) ccw
  circle A9 centre (4.5352, -6.9578) radius 1.525
  arc A10 (7.0381, -5.3039) -> (3.9881, -4.0081) centre (4.5352, -6.9578) ccw
  circle A11 centre (13.5552, -3.9578) radius 1.525
  arc A12 (16.5551, -3.9394) -> (10.5553, -3.9763) centre (13.5552, -3.9578) ccw
  circle A13 centre (-32.018, 29.1502) radius 1.525
  circle A14 centre (-32.018, 9.1502) radius 1.525
  circle A15 centre (-32.018, 19.1502) radius 1.525
  circle A16 centre (-32.018, 39.1502) radius 1.525
  circle A17 centre (11.8181, 24.1899) radius 1.525
  circle A18 centre (-32.018, 49.1502) radius 1.525
  circle A19 centre (11.8203, 44.0353) radius 1.525
  circle A20 centre (11.8205, 34.029) radius 1.525
  line L3 (19.5498, 47.9758) -> (19.8553, 47.9759)
  arc A21 (19.5498, 47.9758) -> (6.5778, 60.1235) centre (6.5778, 47.1235) ccw
  line L4 (-21.2217, 60.1235) -> (6.5778, 60.1235)
  arc A22 (-21.2217, 60.1235) -> (-36.0278, 52.8993) centre (-22.1037, 43.1464) ccw
  line L5 (-40.0187, 52.8985) -> (-36.0278, 52.8993)
  arc A23 (-40.0187, 52.8985) -> (-41.6972, 45.7955) centre (-40.018, 49.1485) ccw
  line L6 (-39.0815, 45.7888) -> (-41.6972, 45.7955)
  arc A24 (-39.0815, 42.7388) -> (-39.0815, 45.7888) centre (-39.0815, 44.2638) ccw
  line L7 (-41.123, 42.732) -> (-39.0815, 42.7388)
  arc A25 (-41.123, 42.732) -> (-41.4471, 35.6815) centre (-40.018, 39.1485) ccw
  line L8 (-39.1197, 35.674) -> (-41.4471, 35.6815)
  arc A26 (-39.1197, 32.624) -> (-39.1197, 35.674) centre (-39.1197, 34.149) ccw
  line L9 (-41.4481, 32.6151) -> (-39.1197, 32.624)
  arc A27 (-41.4481, 32.6151) -> (-41.4504, 25.6829) centre (-40.018, 29.1485) ccw
  line L10 (-39.1197, 25.674) -> (-41.4504, 25.6829)
  arc A28 (-39.1197, 22.624) -> (-39.1197, 25.674) centre (-39.1197, 24.149) ccw
  line L11 (-41.4513, 22.6138) -> (-39.1197, 22.624)
  arc A29 (-41.4513, 22.6138) -> (-41.4536, 15.6842) centre (-40.018, 19.1485) ccw
  line L12 (-39.1197, 15.674) -> (-41.4536, 15.6842)
  arc A30 (-39.1197, 12.624) -> (-39.1197, 15.674) centre (-39.1197, 14.149) ccw
  line L13 (-41.4536, 12.6128) -> (-39.1197, 12.624)
  arc A31 (-41.4536, 12.6128) -> (-40.1195, 5.3999) centre (-40.018, 9.1485) ccw
  line L14 (-39.1197, 5.399) -> (-40.1195, 5.3999)
  line L15 (-39.1197, 2.2457) -> (-39.1197, 5.399)
  arc A32 (-39.1197, 2.2457) -> (-27.0619, -10.7543) centre (-26.1198, 2.2115) ccw
  line L16 (6.5778, -10.7543) -> (-27.0619, -10.7543)
  arc A33 (6.5778, -10.7543) -> (19.5778, 2.2457) centre (6.5778, 2.2457) ccw
  line L17 (19.5778, 10.4758) -> (19.5778, 2.2457)
  line L18 (19.6718, 10.4789) -> (19.5778, 10.4758)
  arc A34 (19.6718, 10.4789) -> (21.251, 17.6915) centre (19.818, 14.2261) ccw
  line L19 (19.5778, 17.7008) -> (21.251, 17.6915)
  arc A35 (19.5778, 20.7508) -> (19.5778, 17.7008) centre (19.5778, 19.2258) ccw
  line L20 (21.2434, 20.7575) -> (19.5778, 20.7508)
  arc A36 (21.2434, 20.7575) -> (21.245, 27.694) centre (19.818, 24.2261) ccw
  line L21 (19.5778, 27.7008) -> (21.245, 27.694)
  arc A37 (19.5778, 30.7508) -> (19.5778, 27.7008) centre (19.5778, 29.2258) ccw
  line L22 (21.2387, 30.7556) -> (19.5778, 30.7508)
  arc A38 (21.2387, 30.7556) -> (21.2402, 37.6959) centre (19.818, 34.2261) ccw
  line L23 (19.5778, 37.7008) -> (21.2402, 37.6959)
  arc A39 (19.5778, 40.7508) -> (19.5778, 37.7008) centre (19.5778, 39.2258) ccw
  line L24 (21.2354, 40.7542) -> (19.5778, 40.7508)
  arc A40 (21.2354, 40.7542) -> (19.8553, 47.9759) centre (19.818, 44.2261) ccw
  circle A41 centre (-11.7277, 35.4153) radius 1.525
  arc A42 (-10.226, 35.6807) -> (-13.1178, 34.7881) centre (-11.7277, 35.4153) ccw
  circle A43 centre (13.563, 14.156) radius 1.525
  arc A44 (13.563, 12.631) -> (13.563, 15.681) centre (13.563, 14.156) ccw
  line L25 (15.088, -1.379) -> (15.088, 16.656)
  point P0 (-17.9415, -10.7543)
  point P1 (-8.4415, -10.7543)
  point P2 (1.5585, -10.7543)
  dimension "d176" = 3.05
  dimension "d177" = 3.05
  dimension "d178" = 3.05
  dimension "d179" = 3.05
  constraint midpoint A0.centre L0
  constraint coincident A0 P0
  constraint midpoint A1.centre L1
  constraint coincident A1 P1
  constraint midpoint A2.centre L2
  constraint coincident A2 P2
  constraint midpoint A3.centre A4
  constraint concentric A5 A6
  constraint concentric A7 A8
  constraint concentric A9 A10
  constraint concentric A11 A12
  constraint concentric A41 A42
  constraint concentric A43 A44
  constraint tangent A43 L25
  measures "d176" diameter of A5
  measures "d177" diameter of A7
  measures "d178" diameter of A9
  measures "d179" diameter of A11
extrude "Extrude27" add sketch "Sketch29" against normal blind 8.7 contours A0 L0 L16 | A1 L1 L16 | A2 L2 L16 | A3 A4 A33 | A3 A4 A33 picked at (-19.7132, -11.3289) picked at (-10.0616, -11.323) picked at (-0.8937, -11.6935) bodies 1
extrude "Extrude28" cut sketch "Sketch29" against normal blind 8.7 contours A5 | A7 | A9 | A11 bodies 1
extrude "Extrude29" cut sketch "BluetoothTop" against normal blind 8.7 contours A8 L18 A10 | L18 A10 bodies 1
copy_body "CopyPasteBodies1" bodies 1 makes body 36
move_body "Move5" bodies 36 to x (1, 0, 0) y (0, 1, 0) z (0, 0, 1) at (155, 0, 0)
move_body "Move6" bodies 36 to x (-1, 0, 0) y (0, 1, 0) z (0, 0, -1) at (0, 0, 0)
move_body "Move7" bodies 36 to x (1, 0, 0) y (0, 1, 0) z (0, 0, 1) at (0, 0, -18)
extrude "Extrude30" add sketch "Sketch29" 7 faces at (3.6136, 30.0188, 0) (-22.6427, 35.155, 0) (-20.2621, -6.8873, 0) (-33.9323, 2.4515, 0) (-25.4617, 54.9573, 0) (-24.242, 25.3452, 0) (11.0144, 8.03, 0) against normal blind 8.7 separate body on bodies 1 makes body 37
move_body "Move21" bodies 37 to x (1, 0, 0) y (0, 1, 0) z (0, 0, 1) at (130, 0, 0)
copy_body "CopyPasteBodies3" bodies 37 makes body 38
move_body "Move22" bodies 38 to x (-1, 0, 0) y (0, 1, 0) z (0, 0, -1) at (-147.536, 0, -17.4)
equation "WoodHeight = 8.7 mm"
equation "PinHeight = 5 mm"
equation "BitSmallSize = 0.9 mm"
equation "HalfBitSize = BitSmallSize / 2"
equation "d5 = -WoodHeight"
equation "ClassicBit = 3 mm"
equation "ClassicBitMarge = ClassicBit + 0.05 mm"
equation "d9 = ClassicBitMarge"
equation "d10 = ClassicBitMarge"
equation "d11 = ClassicBitMarge"
equation "d12 = ClassicBitMarge"
equation "d13 = ClassicBitMarge"
equation "d14 = ClassicBitMarge"
equation "d15 = ClassicBitMarge"
equation "d17 = ClassicBitMarge"
equation "d18 = ClassicBitMarge"
equation "d21 = ClassicBitMarge"
equation "d22 = BitSmallSize"
equation "d23 = -RequiredPinDepth - 1 mm"
equation "d28 = DownTunnelDepth"
equation "d32 = -WoodHeight"
equation "d33 = -WoodHeight"
equation "d35 = -WoodHeight"
equation "d39 = d38"
equation "d40 = d38"
equation "d41 = -RequiredPinDepth - 1 mm"
equation "d43 = DownTunnelDepth"
equation "d47 = -WoodHeight"
equation "JoinLenght = 8 mm"
equation "JoinSize = 7.5 mm"
equation "d51 = JoinLenght"